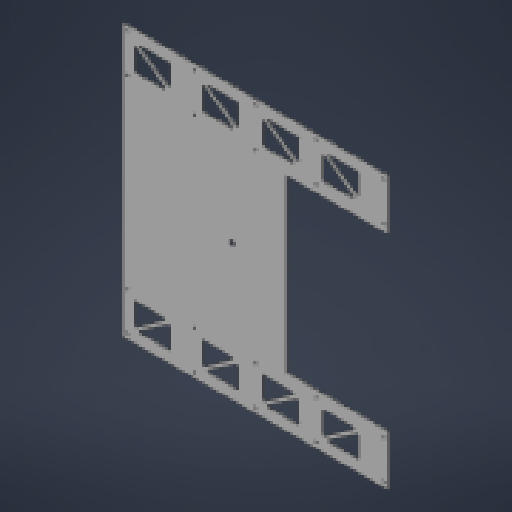
# Autodesk Inventor part: ВЕРХ 25-26
Saved by Autodesk Inventor 2026.2 (Build 302298000, 298)
## iProperties
Created: 2025-09-28
Part Number: ВЕРХ 25-26
Material: Типовые
Document SubType Name: Modeling
Designer: GameHD
Density: 1 g/cm^3
Appearance: По умолчанию
Author: GameHD
Autodesk Inventor part; units mm, degrees
ref_plane "YZ Plane" through (0, 0, 0) normal (1, 0, 0) x (0, 1, 0)
ref_plane "XZ Plane" through (0, 0, 0) normal (0, 1, 0) x (-1, 0, 0)
ref_plane "XY Plane" through (0, 0, 0) normal (0, 0, 1) x (1, 0, 0)
sketch "Эскиз1" plane through (0, 0, 0) normal (0, 0, 1) x (1, 0, 0)
  line L0 (0, 0) -> (380, 0)
  line L1 (380, 0) -> (380, 390)
  line L2 (380, 390) -> (0, 390)
  line L3 (0, 390) -> (0, 0)
  circle A0 centre (189.9999, 7.5) radius 1.625
  circle A1 centre (276.4236, 7.5) radius 1.625
  circle A2 centre (103.5763, 7.5) radius 1.625
  circle A3 centre (373.8998, 7.5) radius 1.625
  circle A4 centre (6.1, 7.5) radius 1.625
  circle A5 centre (964.1922, -67.5828) radius 2.1
  arc A6 (951.6923, -3.9328) -> (946.6923, -8.9328) centre (951.6923, -8.9328) ccw
  line L4 (0, -31.725) -> (0, 41.275)
  line L5 (1326.6922, -81.9328) -> (946.6923, -81.9328)
  line L6 (1326.6922, -8.9328) -> (1326.6922, -81.9328)
  arc A7 (1326.6922, -8.9328) -> (1321.6922, -3.9328) centre (1321.6922, -8.9328) ccw
  line L7 (951.6923, -3.9328) -> (1321.6922, -3.9328)
  line L8 (1216.76, -45.3471) -> (1194.7481, -38.048)
  arc A8 (1220.1863, -50.093) -> (1216.76, -45.3471) centre (1215.1863, -50.093) ccw
  line L9 (1220.1863, -56.3474) -> (1220.1863, -50.093)
  arc A9 (1215.4065, -61.3426) -> (1220.1863, -56.3474) centre (1215.1863, -56.3474) ccw
  line L10 (1169.4571, -63.3681) -> (1215.4065, -61.3426)
  arc A10 (1167.2037, -58.2497) -> (1169.4571, -63.3681) centre (1169.325, -60.3711) ccw
  line L11 (1187.1864, -40.5343) -> (1167.2037, -58.2497)
  arc A11 (1188.5574, -40.0313) -> (1187.1864, -40.5343) centre (1188.5132, -42.0308) ccw
  arc A12 (1188.5574, -40.0313) -> (1192.7788, -38.4615) centre (1188.6922, -33.9328) ccw
  arc A13 (1194.7481, -38.048) -> (1192.7788, -38.4615) centre (1194.1187, -39.9464) ccw
  circle A14 centre (1242.1863, -55.1828) radius 2.15
  circle A15 centre (1226.1863, -55.1828) radius 2.15
  circle A16 centre (1031.1982, -55.1828) radius 2.15
  line L12 (1053.1982, -50.093) -> (1053.1982, -56.3474)
  arc A17 (1056.6245, -45.3471) -> (1053.1982, -50.093) centre (1058.1982, -50.093) ccw
  line L13 (1078.6364, -38.048) -> (1056.6245, -45.3471)
  arc A18 (1080.6057, -38.4615) -> (1078.6364, -38.048) centre (1079.2659, -39.9464) ccw
  arc A19 (1080.6057, -38.4615) -> (1085.5622, -39.9705) centre (1084.6923, -33.9328) ccw
  line L14 (1106.1809, -58.2497) -> (1085.5622, -39.9705)
  arc A20 (1103.9274, -63.3681) -> (1106.1809, -58.2497) centre (1104.0595, -60.3711) ccw
  line L15 (1057.978, -61.3426) -> (1103.9274, -63.3681)
  arc A21 (1053.1982, -56.3474) -> (1057.978, -61.3426) centre (1058.1982, -56.3474) ccw
  circle A22 centre (1047.1982, -55.1828) radius 2.15
  circle A23 centre (1031.1982, -71.1828) radius 2.15
  circle A24 centre (1242.1863, -71.1828) radius 2.15
  circle A25 centre (1093.6922, -74.4328) radius 1.625
  circle A26 centre (1226.1863, -71.1828) radius 2.15
  circle A27 centre (1047.1982, -71.1828) radius 2.15
  circle A28 centre (1154.6923, -73.9328) radius 3.1
  line L16 (1209.2141, -15.9328) -> (1158.2349, -15.9328)
  arc A29 (1209.4653, -16.8651) -> (1209.2141, -15.9328) centre (1209.2141, -16.4328) ccw
  line L17 (1190.2429, -28.0332) -> (1209.4653, -16.8651)
  arc A30 (1190.2429, -28.0332) -> (1184.8228, -29.2171) centre (1188.6922, -33.9328) ccw
  arc A31 (1182.8362, -29.5377) -> (1184.8228, -29.2171) centre (1183.5541, -27.671) ccw
  line L18 (1157.517, -19.7995) -> (1182.8362, -29.5377)
  arc A32 (1158.2349, -15.9328) -> (1157.517, -19.7995) centre (1158.2349, -17.9328) ccw
  line L19 (1063.9192, -16.8651) -> (1083.1416, -28.0332)
  arc A33 (1064.1704, -15.9328) -> (1063.9192, -16.8651) centre (1064.1704, -16.4328) ccw
  line L20 (1115.1496, -15.9328) -> (1064.1704, -15.9328)
  arc A34 (1115.8675, -19.7995) -> (1115.1496, -15.9328) centre (1115.1496, -17.9328) ccw
  line L21 (1090.5483, -29.5377) -> (1115.8675, -19.7995)
  arc A35 (1088.5617, -29.2171) -> (1090.5483, -29.5377) centre (1089.8304, -27.671) ccw
  arc A36 (1088.5617, -29.2171) -> (1083.1416, -28.0332) centre (1084.6923, -33.9328) ccw
  line L22 (1110.9153, -57.1805) -> (1113.5672, -59.5315)
  arc A37 (1110.6057, -54.534) -> (1110.9153, -57.1805) centre (1112.2421, -55.6839) ccw
  line L23 (1131.0559, -25.4322) -> (1110.6057, -54.534)
  arc A38 (1134.6923, -26.5821) -> (1131.0559, -25.4322) centre (1132.6923, -26.5821) ccw
  line L24 (1134.6923, -61.3681) -> (1134.6923, -26.5821)
  arc A39 (1132.6923, -63.3681) -> (1134.6923, -61.3681) centre (1132.6923, -61.3681) ccw
  line L25 (1123.3837, -63.3681) -> (1132.6923, -63.3681)
  arc A40 (1121.7315, -62.4952) -> (1123.3837, -63.3681) centre (1123.3837, -61.3681) ccw
  arc A41 (1121.7315, -62.4952) -> (1115.338, -59.985) centre (1116.6923, -65.9328) ccw
  arc A42 (1113.5672, -59.5315) -> (1115.338, -59.985) centre (1114.894, -58.035) ccw
  line L26 (1168.4937, -51.8395) -> (1182.0952, -39.7813)
  arc A43 (1165.5306, -51.4929) -> (1168.4937, -51.8395) centre (1167.167, -50.343) ccw
  line L27 (1145.8825, -23.5324) -> (1165.5306, -51.4929)
  arc A44 (1148.2368, -20.5158) -> (1145.8825, -23.5324) centre (1147.5188, -22.3825) ccw
  line L28 (1180.7096, -33.0054) -> (1148.2368, -20.5158)
  arc A45 (1182.096, -34.0931) -> (1180.7096, -33.0054) centre (1179.6327, -35.8054) ccw
  arc A46 (1182.7689, -35.3904) -> (1182.096, -34.0931) centre (1177.4301, -37.3365) ccw
  arc A47 (1182.7689, -35.3904) -> (1182.9531, -35.9999) centre (1188.6922, -33.9328) ccw
  arc A48 (1183.0967, -37.7601) -> (1182.9531, -35.9999) centre (1177.4301, -37.3365) ccw
  arc A49 (1182.0952, -39.7813) -> (1183.0967, -37.7601) centre (1180.105, -37.5364) ccw
  line L29 (1125.1477, -20.5158) -> (1092.6749, -33.0054)
  arc A50 (1127.5021, -23.5324) -> (1125.1477, -20.5158) centre (1125.8657, -22.3825) ccw
  line L30 (1107.8539, -51.4929) -> (1127.5021, -23.5324)
  arc A51 (1104.8908, -51.8395) -> (1107.8539, -51.4929) centre (1106.2176, -50.343) ccw
  line L31 (1091.2893, -39.7813) -> (1104.8908, -51.8395)
  arc A52 (1090.2878, -37.7601) -> (1091.2893, -39.7813) centre (1093.2795, -37.5364) ccw
  arc A53 (1090.4314, -35.9999) -> (1090.2878, -37.7601) centre (1095.9544, -37.3365) ccw
  arc A54 (1090.4314, -35.9999) -> (1090.6156, -35.3904) centre (1084.6923, -33.9328) ccw
  arc A55 (1091.2885, -34.0931) -> (1090.6156, -35.3904) centre (1095.9544, -37.3365) ccw
  arc A56 (1092.6749, -33.0054) -> (1091.2885, -34.0931) centre (1093.7519, -35.8054) ccw
  line L32 (1162.7788, -54.534) -> (1142.3286, -25.4322)
  arc A57 (1162.4692, -57.1805) -> (1162.7788, -54.534) centre (1161.1424, -55.6839) ccw
  line L33 (1156.0575, -62.8647) -> (1162.4692, -57.1805)
  arc A58 (1154.7308, -63.3681) -> (1156.0575, -62.8647) centre (1154.7308, -61.3681) ccw
  line L34 (1140.6923, -63.3681) -> (1154.7308, -63.3681)
  arc A59 (1138.6923, -61.3681) -> (1140.6923, -63.3681) centre (1140.6923, -61.3681) ccw
  line L35 (1138.6923, -26.5821) -> (1138.6923, -61.3681)
  arc A60 (1142.3286, -25.4322) -> (1138.6923, -26.5821) centre (1140.6923, -26.5821) ccw
  arc A61 (1252.9105, -48.8923) -> (1251.6365, -50.9573) centre (1270.1159, -60.9328) ccw
  arc A62 (1249.247, -51.9056) -> (1251.6365, -50.9573) centre (1249.8765, -50.0073) ccw
  line L36 (1197.3221, -34.6874) -> (1249.247, -51.9056)
  arc A63 (1196.7592, -29.2459) -> (1197.3221, -34.6874) centre (1198.2663, -31.8398) ccw
  line L37 (1216.329, -17.8759) -> (1196.7592, -29.2459)
  arc A64 (1218.7614, -18.2046) -> (1216.329, -17.8759) centre (1217.3337, -19.6052) ccw
  arc A65 (1218.7614, -18.2046) -> (1224.7366, -19.8136) centre (1223.1159, -13.9328) ccw
  arc A66 (1226.6821, -20.3275) -> (1224.7366, -19.8136) centre (1225.2679, -21.7417) ccw
  line L38 (1252.6861, -46.3314) -> (1226.6821, -20.3275)
  arc A67 (1252.9105, -48.8923) -> (1252.6861, -46.3314) centre (1251.2719, -47.7456) ccw
  arc A68 (1048.648, -19.8136) -> (1054.6231, -18.2046) centre (1050.2686, -13.9328) ccw
  arc A69 (1057.0555, -17.8759) -> (1054.6231, -18.2046) centre (1056.0508, -19.6052) ccw
  line L39 (1076.6253, -29.2459) -> (1057.0555, -17.8759)
  arc A70 (1076.0624, -34.6874) -> (1076.6253, -29.2459) centre (1075.1182, -31.8398) ccw
  line L40 (1024.1375, -51.9056) -> (1076.0624, -34.6874)
  arc A71 (1021.7481, -50.9573) -> (1024.1375, -51.9056) centre (1023.508, -50.0073) ccw
  arc A72 (1021.7481, -50.9573) -> (1020.4741, -48.8923) centre (1003.2686, -60.9328) ccw
  arc A73 (1020.6985, -46.3314) -> (1020.4741, -48.8923) centre (1022.1127, -47.7456) ccw
  line L41 (1046.7024, -20.3275) -> (1020.6985, -46.3314)
  arc A74 (1048.648, -19.8136) -> (1046.7024, -20.3275) centre (1048.1166, -21.7417) ccw
  circle A75 centre (1039.1982, -63.1828) radius 6
  circle A76 centre (1234.1863, -63.1828) radius 6
  arc A77 (1291.0993, -61.7677) -> (1287.7395, -49.5132) centre (1270.1159, -60.9328) ccw
  arc A78 (1288.0551, -46.9619) -> (1287.7395, -49.5132) centre (1289.418, -48.4256) ccw
  line L42 (1313.5478, -23.2248) -> (1288.0551, -46.9619)
  arc A79 (1318.5922, -25.4204) -> (1313.5478, -23.2248) centre (1315.5922, -25.4204) ccw
  line L43 (1318.5922, -64.0897) -> (1318.5922, -25.4204)
  arc A80 (1318.0461, -65.8154) -> (1318.5922, -64.0897) centre (1315.5922, -64.0897) ccw
  arc A81 (1315.1572, -68.1426) -> (1318.0461, -65.8154) centre (1312.5518, -61.9515) ccw
  arc A82 (1313.3548, -68.3086) -> (1315.1572, -68.1426) centre (1313.9935, -65.3774) ccw
  line L44 (1292.6719, -63.8013) -> (1313.3548, -68.3086)
  arc A83 (1291.0993, -61.7677) -> (1292.6719, -63.8013) centre (1293.0977, -61.8472) ccw
  arc A84 (1015.3091, -43.7274) -> (990.6226, -44.1674) centre (1003.2686, -60.9328) ccw
  arc A85 (988.0553, -44.0344) -> (990.6226, -44.1674) centre (989.4182, -42.5707) ccw
  line L45 (963.455, -21.1284) -> (988.0553, -44.0344)
  arc A86 (965.4994, -15.9328) -> (963.455, -21.1284) centre (965.4994, -18.9328) ccw
  line L46 (1043.026, -15.9328) -> (965.4994, -15.9328)
  arc A87 (1043.7331, -17.6399) -> (1043.026, -15.9328) centre (1043.026, -16.9328) ccw
  line L47 (1017.87, -43.503) -> (1043.7331, -17.6399)
  arc A88 (1015.3091, -43.7274) -> (1017.87, -43.503) centre (1016.4558, -42.0887) ccw
  line L48 (1229.6514, -17.6399) -> (1255.5145, -43.503)
  arc A89 (1230.3585, -15.9328) -> (1229.6514, -17.6399) centre (1230.3585, -16.9328) ccw
  line L49 (1307.8851, -15.9328) -> (1230.3585, -15.9328)
  arc A90 (1309.9295, -21.1284) -> (1307.8851, -15.9328) centre (1307.8851, -18.9328) ccw
  line L50 (1285.3292, -44.0344) -> (1309.9295, -21.1284)
  arc A91 (1282.7619, -44.1674) -> (1285.3292, -44.0344) centre (1283.9663, -42.5707) ccw
  arc A92 (1282.7619, -44.1674) -> (1258.0754, -43.7274) centre (1270.1159, -60.9328) ccw
  arc A93 (1255.5145, -43.503) -> (1258.0754, -43.7274) centre (1256.9287, -42.0887) ccw
  circle A94 centre (1319.6922, -74.4328) radius 1.625
  circle A95 centre (953.6923, -74.4328) radius 1.625
  circle A96 centre (1179.6922, -74.4328) radius 1.625
  circle A97 centre (1084.6923, -33.9328) radius 2.1
  circle A98 centre (1116.6923, -65.9328) radius 2.1
  circle A99 centre (1003.2686, -60.9328) radius 4
  circle A100 centre (994.2686, -60.9328) radius 2.1
  circle A101 centre (1279.1159, -60.9328) radius 2.1
  circle A102 centre (1270.1159, -69.9328) radius 2.1
  circle A103 centre (1270.1159, -60.9328) radius 4
  circle A104 centre (1003.2686, -51.9328) radius 2.1
  circle A105 centre (1003.2686, -69.9328) radius 2.1
  circle A106 centre (1012.2686, -60.9328) radius 2.1
  circle A107 centre (1270.1159, -51.9328) radius 2.1
  circle A108 centre (1261.1159, -60.9328) radius 2.1
  arc A109 (969.1578, -64.2135) -> (967.1922, -62.5828) centre (967.1922, -64.5828) ccw
  line L51 (967.1922, -62.5828) -> (956.7923, -62.5828)
  arc A110 (954.7923, -60.5828) -> (956.7923, -62.5828) centre (956.7923, -60.5828) ccw
  line L52 (954.7923, -25.4204) -> (954.7923, -60.5828)
  arc A111 (959.8367, -23.2248) -> (954.7923, -25.4204) centre (957.7923, -25.4204) ccw
  line L53 (985.3295, -46.9619) -> (959.8367, -23.2248)
  arc A112 (985.645, -49.5132) -> (985.3295, -46.9619) centre (983.9666, -48.4256) ccw
  arc A113 (985.645, -49.5132) -> (982.2852, -61.7677) centre (1003.2686, -60.9328) ccw
  arc A114 (980.7127, -63.8013) -> (982.2852, -61.7677) centre (980.2868, -61.8472) ccw
  line L54 (971.5492, -65.7983) -> (980.7127, -63.8013)
  arc A115 (969.1578, -64.2135) -> (971.5492, -65.7983) centre (971.1234, -63.8441) ccw
  line L55 (0, 195) -> (417.5125, 195)
  circle A116 centre (189.9999, 382.5) radius 1.625
  circle A117 centre (276.4236, 382.5) radius 1.625
  circle A118 centre (373.8998, 382.5) radius 1.625
  circle A119 centre (103.5763, 382.5) radius 1.625
  circle A120 centre (6.1, 382.5) radius 1.625
  line L56 (-36.5125, 35) -> (652.4625, 35)
  circle A121 centre (189.9999, 62.5) radius 1.625
  circle A122 centre (276.4236, 62.5) radius 1.625
  circle A123 centre (373.8998, 62.5) radius 1.625
  circle A124 centre (103.5763, 62.5) radius 1.625
  circle A125 centre (6.1, 62.5) radius 1.625
  circle A126 centre (189.9999, 327.5) radius 1.625
  circle A127 centre (103.5763, 327.5) radius 1.625
  circle A128 centre (373.8998, 327.5) radius 1.625
  circle A129 centre (6.1, 327.5) radius 1.625
  circle A130 centre (276.4236, 327.5) radius 1.625
  line L57 (380, 195) -> (280, 195)
  line L58 (280, 195) -> (280, 73)
  line L59 (280, 73) -> (380, 73)
  line L60 (380, 73) -> (380, 195)
  line L61 (280, 195) -> (280, 317)
  line L62 (280, 317) -> (380, 317)
  point P0 (1137.8297, -60.6207)
  point P1 (0, 348.725)
  dimension "d0" = 380
  dimension "d1" = 390
  dimension "d2" = 7.5
  dimension "d3" = 0
  dimension "d4" = 0
  dimension "d5" = 0
  dimension "d6" = 0
  dimension "d7" = 35
  dimension "d8" = 100
  dimension "d9" = 122
  constraints: 166 point on circle, 131 centre point, 126 end point, 18 symmetric about line, 4 horizontal, 4 parallel, 2 midpoint, 2 perpendicular, 1 point on line, 15 other
  measures "d0" distance of L2.end L1.end
  measures "d1" distance of L1.end L0.end
  measures "d2" distance from line of L0 A4.centre
  measures "d3" vertical distance of A4.centre A2.centre
  measures "d4" vertical distance of A2.centre A0.centre
  measures "d5" vertical distance of A0.centre A1.centre
  measures "d6" vertical distance of A1.centre A3.centre
  measures "d7" distance between parallel lines of L0 L56
  measures "d8" distance of L59.end L58.end
  measures "d9" distance of L58.end L57.end
extrude "Выдавливание1" add sketch "Эскиз1" along normal blind 1.5 contours L3 L56 L1 L0 | L3 L55 L58 L59 L1 L56 | L3 L2 L1 L62 L61 L55
sketch "Эскиз2" plane through (0, 0, 1.5) normal (0, 0, 1) x (1, 0, 0)
  line L0 (25.7748, 373.5) -> (65.85, 373.5)
  arc A0 (67.85, 371.5) -> (65.85, 373.5) centre (65.85, 371.5) ccw
  arc A1 (25.7748, 373.5) -> (24.6115, 369.8731) centre (25.7748, 371.5) ccw
  arc A2 (19.2632, 368.7798) -> (16.1, 367.1528) centre (18.1, 367.1528) ccw
  line L1 (67.85, 371.5) -> (67.85, 344.5882)
  line L2 (64.6868, 342.9612) -> (24.6115, 369.8731)
  line L3 (67.85, 336.5) -> (16.1, 373.5)
  arc A3 (58.1752, 336.5) -> (59.3385, 340.1269) centre (58.1752, 338.5) ccw
  arc A4 (64.6868, 342.9612) -> (67.85, 344.5882) centre (65.85, 344.5882) ccw
  line L4 (58.1752, 336.5) -> (18.1, 336.5)
  line L5 (16.1, 338.5) -> (16.1, 367.1528)
  arc A5 (16.1, 338.5) -> (18.1, 336.5) centre (18.1, 338.5) ccw
  line L6 (59.3385, 340.1269) -> (19.2632, 368.7798)
  circle A6 centre (6.1, 382.5) radius 1.625 projected
  line L7 (280, 73) -> (280, 317) projected
  line L8 (280, 317) -> (380, 317) projected
  line L9 (380, 317) -> (380, 390) projected
  line L10 (380, 390) -> (0, 390) projected
  line L11 (0, 390) -> (0, 0) projected
  line L12 (0, 0) -> (380, 0) projected
  line L13 (380, 0) -> (380, 73) projected
  line L14 (380, 73) -> (280, 73) projected
  circle A7 centre (373.8998, 327.5) radius 1.625 projected
  circle A8 centre (189.9999, 327.5) radius 1.625 projected
  circle A9 centre (6.1, 327.5) radius 1.625 projected
  circle A10 centre (103.5763, 382.5) radius 1.625 projected
  circle A11 centre (276.4236, 382.5) radius 1.625 projected
  circle A12 centre (189.9999, 382.5) radius 1.625 projected
  circle A13 centre (373.8998, 382.5) radius 1.625 projected
  circle A14 centre (6.1, 382.5) radius 1.625 projected
  circle A15 centre (103.5763, 327.5) radius 1.625 projected
  circle A16 centre (276.4236, 327.5) radius 1.625 projected
  circle A17 centre (103.5763, 7.5) radius 1.625 projected
  circle A18 centre (373.8998, 7.5) radius 1.625 projected
  circle A19 centre (276.4236, 7.5) radius 1.625 projected
  circle A20 centre (189.9999, 7.5) radius 1.625 projected
  circle A21 centre (6.1, 7.5) radius 1.625 projected
  circle A22 centre (189.9999, 62.5) radius 1.625 projected
  circle A23 centre (103.5763, 62.5) radius 1.625 projected
  circle A24 centre (373.8998, 62.5) radius 1.625 projected
  circle A25 centre (6.1, 62.5) radius 1.625 projected
  circle A26 centre (276.4236, 62.5) radius 1.625 projected
  arc A27 (123.251, 373.5) -> (122.0878, 369.8731) centre (123.251, 371.5) ccw
  arc A28 (116.7395, 368.7798) -> (113.5763, 367.1528) centre (115.5763, 367.1528) ccw
  line L15 (113.5763, 338.5) -> (113.5763, 367.1528)
  arc A29 (113.5763, 338.5) -> (115.5763, 336.5) centre (115.5763, 338.5) ccw
  line L16 (123.251, 373.5) -> (163.3263, 373.5)
  line L17 (156.8147, 340.1269) -> (116.7395, 368.7798)
  line L18 (155.6515, 336.5) -> (115.5763, 336.5)
  line L19 (165.3263, 336.5) -> (113.5763, 373.5)
  line L20 (162.1631, 342.9612) -> (122.0878, 369.8731)
  arc A30 (165.3263, 371.5) -> (163.3263, 373.5) centre (163.3263, 371.5) ccw
  line L21 (165.3263, 371.5) -> (165.3263, 344.5882)
  arc A31 (155.6515, 336.5) -> (156.8147, 340.1269) centre (155.6515, 338.5) ccw
  arc A32 (162.1631, 342.9612) -> (165.3263, 344.5882) centre (163.3263, 344.5882) ccw
  arc A33 (209.6747, 373.5) -> (208.5115, 369.8731) centre (209.6747, 371.5) ccw
  arc A34 (203.1631, 368.7798) -> (199.9999, 367.1528) centre (201.9999, 367.1528) ccw
  line L22 (199.9999, 338.5) -> (199.9999, 367.1528)
  arc A35 (199.9999, 338.5) -> (201.9999, 336.5) centre (201.9999, 338.5) ccw
  line L23 (209.6747, 373.5) -> (249.7499, 373.5)
  line L24 (243.2384, 340.1269) -> (203.1631, 368.7798)
  line L25 (242.0752, 336.5) -> (201.9999, 336.5)
  line L26 (251.7499, 336.5) -> (199.9999, 373.5)
  line L27 (248.5867, 342.9612) -> (208.5115, 369.8731)
  arc A36 (251.7499, 371.5) -> (249.7499, 373.5) centre (249.7499, 371.5) ccw
  line L28 (251.7499, 371.5) -> (251.7499, 344.5882)
  arc A37 (242.0752, 336.5) -> (243.2384, 340.1269) centre (242.0752, 338.5) ccw
  arc A38 (248.5867, 342.9612) -> (251.7499, 344.5882) centre (249.7499, 344.5882) ccw
  arc A39 (296.0983, 373.5) -> (294.9351, 369.8731) centre (296.0983, 371.5) ccw
  arc A40 (289.5868, 368.7798) -> (286.4236, 367.1528) centre (288.4236, 367.1528) ccw
  line L29 (286.4236, 338.5) -> (286.4236, 367.1528)
  arc A41 (286.4236, 338.5) -> (288.4236, 336.5) centre (288.4236, 338.5) ccw
  line L30 (296.0983, 373.5) -> (336.1736, 373.5)
  line L31 (329.662, 340.1269) -> (289.5868, 368.7798)
  line L32 (328.4988, 336.5) -> (288.4236, 336.5)
  line L33 (338.1736, 336.5) -> (286.4236, 373.5)
  line L34 (335.0103, 342.9612) -> (294.9351, 369.8731)
  arc A42 (338.1736, 371.5) -> (336.1736, 373.5) centre (336.1736, 371.5) ccw
  line L35 (338.1736, 371.5) -> (338.1736, 344.5882)
  arc A43 (328.4988, 336.5) -> (329.662, 340.1269) centre (328.4988, 338.5) ccw
  arc A44 (335.0103, 342.9612) -> (338.1736, 344.5882) centre (336.1736, 344.5882) ccw
  line L36 (0, 195) -> (395.2875, 195)
  arc A45 (24.6115, 20.1269) -> (25.7748, 16.5) centre (25.7748, 18.5) ccw
  arc A46 (16.1, 22.8472) -> (19.2632, 21.2202) centre (18.1, 22.8472) ccw
  line L37 (16.1, 51.5) -> (16.1, 22.8472)
  arc A47 (18.1, 53.5) -> (16.1, 51.5) centre (18.1, 51.5) ccw
  line L38 (25.7748, 16.5) -> (65.85, 16.5)
  line L39 (59.3385, 49.8731) -> (19.2632, 21.2202)
  line L40 (58.1752, 53.5) -> (18.1, 53.5)
  line L41 (67.85, 53.5) -> (16.1, 16.5)
  line L42 (64.6868, 47.0388) -> (24.6115, 20.1269)
  arc A48 (65.85, 16.5) -> (67.85, 18.5) centre (65.85, 18.5) ccw
  line L43 (67.85, 18.5) -> (67.85, 45.4118)
  arc A49 (59.3385, 49.8731) -> (58.1752, 53.5) centre (58.1752, 51.5) ccw
  arc A50 (67.85, 45.4118) -> (64.6868, 47.0388) centre (65.85, 45.4118) ccw
  line L44 (155.6515, 53.5) -> (115.5763, 53.5)
  line L45 (156.8147, 49.8731) -> (116.7395, 21.2202)
  line L46 (165.3263, 53.5) -> (113.5763, 16.5)
  line L47 (162.1631, 47.0388) -> (122.0878, 20.1269)
  arc A51 (156.8147, 49.8731) -> (155.6515, 53.5) centre (155.6515, 51.5) ccw
  arc A52 (165.3263, 45.4118) -> (162.1631, 47.0388) centre (163.3263, 45.4118) ccw
  line L48 (165.3263, 18.5) -> (165.3263, 45.4118)
  arc A53 (163.3263, 16.5) -> (165.3263, 18.5) centre (163.3263, 18.5) ccw
  line L49 (123.251, 16.5) -> (163.3263, 16.5)
  arc A54 (115.5763, 53.5) -> (113.5763, 51.5) centre (115.5763, 51.5) ccw
  arc A55 (122.0878, 20.1269) -> (123.251, 16.5) centre (123.251, 18.5) ccw
  line L50 (113.5763, 51.5) -> (113.5763, 22.8472)
  arc A56 (113.5763, 22.8472) -> (116.7395, 21.2202) centre (115.5763, 22.8472) ccw
  line L51 (242.0752, 53.5) -> (201.9999, 53.5)
  line L52 (243.2384, 49.8731) -> (203.1631, 21.2202)
  line L53 (251.7499, 53.5) -> (199.9999, 16.5)
  line L54 (248.5867, 47.0388) -> (208.5115, 20.1269)
  arc A57 (243.2384, 49.8731) -> (242.0752, 53.5) centre (242.0752, 51.5) ccw
  arc A58 (251.7499, 45.4118) -> (248.5867, 47.0388) centre (249.7499, 45.4118) ccw
  line L55 (251.7499, 18.5) -> (251.7499, 45.4118)
  arc A59 (249.7499, 16.5) -> (251.7499, 18.5) centre (249.7499, 18.5) ccw
  line L56 (209.6747, 16.5) -> (249.7499, 16.5)
  arc A60 (201.9999, 53.5) -> (199.9999, 51.5) centre (201.9999, 51.5) ccw
  arc A61 (208.5115, 20.1269) -> (209.6747, 16.5) centre (209.6747, 18.5) ccw
  line L57 (199.9999, 51.5) -> (199.9999, 22.8472)
  arc A62 (199.9999, 22.8472) -> (203.1631, 21.2202) centre (201.9999, 22.8472) ccw
  line L58 (328.4988, 53.5) -> (288.4236, 53.5)
  line L59 (329.662, 49.8731) -> (289.5868, 21.2202)
  line L60 (338.1736, 53.5) -> (286.4236, 16.5)
  line L61 (335.0103, 47.0388) -> (294.9351, 20.1269)
  arc A63 (329.662, 49.8731) -> (328.4988, 53.5) centre (328.4988, 51.5) ccw
  arc A64 (338.1736, 45.4118) -> (335.0103, 47.0388) centre (336.1736, 45.4118) ccw
  line L62 (338.1736, 18.5) -> (338.1736, 45.4118)
  arc A65 (336.1736, 16.5) -> (338.1736, 18.5) centre (336.1736, 18.5) ccw
  line L63 (296.0983, 16.5) -> (336.1736, 16.5)
  arc A66 (288.4236, 53.5) -> (286.4236, 51.5) centre (288.4236, 51.5) ccw
  arc A67 (294.9351, 20.1269) -> (296.0983, 16.5) centre (296.0983, 18.5) ccw
  line L64 (286.4236, 51.5) -> (286.4236, 22.8472)
  arc A68 (286.4236, 22.8472) -> (289.5868, 21.2202) centre (288.4236, 22.8472) ccw
  dimension "d12" = 37
  dimension "d13" = 51.75
  dimension "d16" = 10
  dimension "d17" = 9
  dimension "d18" = 47.75
  dimension "d19" = 4.3472
  dimension "d20" = 33
  dimension "d21" = 2
  dimension "d22" = 2
  dimension "d23" = 2
  dimension "d24" = 2
  dimension "d25" = 2
  dimension "d26" = 2
  dimension "d27" = 28.6528
  dimension "d28" = 2
  dimension "d29" = 37
  dimension "d30" = 51.75
  dimension "d31" = 47.75
  dimension "d32" = 4.3472
  dimension "d33" = 33
  dimension "d34" = 2
  dimension "d35" = 2
  dimension "d36" = 2
  dimension "d37" = 2
  dimension "d38" = 2
  dimension "d39" = 2
  dimension "d40" = 28.6528
  dimension "d41" = 2
  dimension "d42" = 37
  dimension "d43" = 51.75
  dimension "d44" = 47.75
  dimension "d45" = 4.3472
  dimension "d46" = 33
  dimension "d47" = 2
  dimension "d48" = 2
  dimension "d49" = 2
  dimension "d50" = 2
  dimension "d51" = 2
  dimension "d52" = 2
  dimension "d53" = 28.6528
  dimension "d54" = 2
  dimension "d55" = 37
  dimension "d56" = 51.75
  dimension "d57" = 47.75
  dimension "d58" = 4.3472
  dimension "d59" = 33
  dimension "d60" = 2
  dimension "d61" = 2
  dimension "d62" = 2
  dimension "d63" = 2
  dimension "d64" = 2
  dimension "d65" = 2
  dimension "d66" = 28.6528
  dimension "d67" = 2
  constraints: 114 end point, 96 point on circle, 80 symmetric about line, 48 centre point, 32 point on line, 1 horizontal, 1 midpoint, 24 other
  measures "d12" distance between parallel lines of L4 L0
  measures "d13" distance between parallel lines of L1 L5
  measures "d16" distance from line of A6.centre L5
  measures "d17" distance from line of A6.centre L0
  measures "d18" horizontal distance of A0.centre A5.centre
  measures "d19" vertical distance of A1.centre A2.centre
  measures "d20" vertical distance of A3.centre A1.centre
  measures "d21" radius of A1
  measures "d22" radius of A2
  measures "d23" radius of A5
  measures "d24" radius of A3
  measures "d25" radius of A0
  measures "d26" radius of A4
  measures "d27" distance of L5.start L5.end
  measures "d28" distance from line of A2.centre L5
  measures "d29" distance between parallel lines of L18 L16
  measures "d30" distance between parallel lines of L21 L15
  measures "d31" horizontal distance of A30.centre A29.centre
  measures "d32" vertical distance of A27.centre A28.centre
  measures "d33" vertical distance of A31.centre A27.centre
  measures "d34" radius of A27
  measures "d35" radius of A28
  measures "d36" radius of A29
  measures "d37" radius of A31
  measures "d38" radius of A30
  measures "d39" radius of A32
  measures "d40" distance of L15.start L15.end
  measures "d41" distance from line of A28.centre L15
  measures "d42" distance between parallel lines of L25 L23
  measures "d43" distance between parallel lines of L28 L22
  measures "d44" horizontal distance of A36.centre A35.centre
  measures "d45" vertical distance of A33.centre A34.centre
  measures "d46" vertical distance of A37.centre A33.centre
  measures "d47" radius of A33
  measures "d48" radius of A34
  measures "d49" radius of A35
  measures "d50" radius of A37
  measures "d51" radius of A36
  measures "d52" radius of A38
  measures "d53" distance of L22.start L22.end
  measures "d54" distance from line of A34.centre L22
  measures "d55" distance between parallel lines of L32 L30
  measures "d56" distance between parallel lines of L35 L29
  measures "d57" horizontal distance of A42.centre A41.centre
  measures "d58" vertical distance of A39.centre A40.centre
  measures "d59" vertical distance of A43.centre A39.centre
  measures "d60" radius of A39
  measures "d61" radius of A40
  measures "d62" radius of A41
  measures "d63" radius of A43
  measures "d64" radius of A42
  measures "d65" radius of A44
  measures "d66" distance of L29.start L29.end
  measures "d67" distance from line of A40.centre L29
extrude "Выдавливание2" cut sketch "Эскиз2" against normal blind 1.5 contours L0 A0 L1 A4 L2 A1 | L6 A3 L4 A5 L5 A2 | L16 A30 L21 A32 L20 A27 | L17 A31 L18 A29 L15 A28 | L23 A36 L28 A38 L27 A33 | L24 A37 L25 A35 L22 A34 | L30 A42 L35 A44 L34 A39 | L31 A43 L32 A41 L29 A40 | L42 A50 L43 A48 L38 A45 | L37 A47 L40 A49 L39 A46 | A51 L45 A56 L50 A54 L44 | A52 L48 A53 L49 A55 L47 | A57 L52 A62 L57 A60 L51 | A58 L55 A59 L56 A61 L54 | A63 L59 A68 L64 A66 L58 | A64 L62 A65 L63 A67 L61
sketch "Эскиз4" plane through (0, 0, 1.5) normal (0, 0, 1) x (1, 0, 0)
  line L0 (391.3464, 129.9271) -> (391.3464, 259.9271) projected
  line L1 (199.3064, 259.9271) -> (391.3464, 259.9271) projected
  line L2 (199.3064, 129.9271) -> (199.3064, 259.9271) projected
  line L3 (391.3464, 129.9271) -> (199.3064, 129.9271) projected
  circle A0 centre (276.4236, 62.5) radius 1.625 projected
  circle A1 centre (6.1, 62.5) radius 1.625 projected
  circle A2 centre (373.8998, 62.5) radius 1.625 projected
  circle A3 centre (103.5763, 62.5) radius 1.625 projected
  circle A4 centre (189.9999, 62.5) radius 1.625 projected
  circle A5 centre (6.1, 7.5) radius 1.625 projected
  circle A6 centre (189.9999, 7.5) radius 1.625 projected
  circle A7 centre (276.4236, 7.5) radius 1.625 projected
  circle A8 centre (373.8998, 7.5) radius 1.625 projected
  circle A9 centre (103.5763, 7.5) radius 1.625 projected
  circle A10 centre (276.4236, 327.5) radius 1.625 projected
  circle A11 centre (103.5763, 327.5) radius 1.625 projected
  circle A12 centre (6.1, 382.5) radius 1.625 projected
  circle A13 centre (373.8998, 382.5) radius 1.625 projected
  circle A14 centre (189.9999, 382.5) radius 1.625 projected
  circle A15 centre (276.4236, 382.5) radius 1.625 projected
  circle A16 centre (103.5763, 382.5) radius 1.625 projected
  circle A17 centre (6.1, 327.5) radius 1.625 projected
  circle A18 centre (189.9999, 327.5) radius 1.625 projected
  circle A19 centre (373.8998, 327.5) radius 1.625 projected
  line L4 (0, 390) -> (0, 0) projected
  line L5 (0, 0) -> (380, 0) projected
  line L6 (380, 0) -> (380, 73) projected
  line L7 (380, 73) -> (280, 73) projected
  line L8 (280, 73) -> (280, 317) projected
  line L9 (280, 317) -> (380, 317) projected
  line L10 (380, 317) -> (380, 390) projected
  line L11 (380, 390) -> (0, 390) projected
  line L12 (67.85, 45.4118) -> (67.85, 18.5) projected
  arc A20 (65.85, 16.5) -> (67.85, 18.5) centre (65.85, 18.5) ccw projected
  line L13 (65.85, 16.5) -> (25.7748, 16.5) projected
  arc A21 (24.6115, 20.1269) -> (25.7748, 16.5) centre (25.7748, 18.5) ccw projected
  line L14 (24.6115, 20.1269) -> (64.6868, 47.0388) projected
  arc A22 (67.85, 45.4118) -> (64.6868, 47.0388) centre (65.85, 45.4118) ccw projected
  arc A23 (201.9999, 53.5) -> (199.9999, 51.5) centre (201.9999, 51.5) ccw projected
  line L15 (201.9999, 53.5) -> (242.0752, 53.5) projected
  arc A24 (243.2384, 49.8731) -> (242.0752, 53.5) centre (242.0752, 51.5) ccw projected
  line L16 (243.2384, 49.8731) -> (203.1631, 21.2202) projected
  arc A25 (199.9999, 22.8472) -> (203.1631, 21.2202) centre (201.9999, 22.8472) ccw projected
  line L17 (199.9999, 22.8472) -> (199.9999, 51.5) projected
  arc A26 (25.7748, 373.5) -> (24.6115, 369.8731) centre (25.7748, 371.5) ccw projected
  line L18 (25.7748, 373.5) -> (65.85, 373.5) projected
  arc A27 (67.85, 371.5) -> (65.85, 373.5) centre (65.85, 371.5) ccw projected
  line L19 (67.85, 371.5) -> (67.85, 344.5882) projected
  arc A28 (64.6868, 342.9612) -> (67.85, 344.5882) centre (65.85, 344.5882) ccw projected
  line L20 (64.6868, 342.9612) -> (24.6115, 369.8731) projected
  line L21 (199.9999, 338.5) -> (199.9999, 367.1528) projected
  arc A29 (203.1631, 368.7798) -> (199.9999, 367.1528) centre (201.9999, 367.1528) ccw projected
  line L22 (203.1631, 368.7798) -> (243.2384, 340.1269) projected
  arc A30 (242.0752, 336.5) -> (243.2384, 340.1269) centre (242.0752, 338.5) ccw projected
  line L23 (242.0752, 336.5) -> (201.9999, 336.5) projected
  arc A31 (199.9999, 338.5) -> (201.9999, 336.5) centre (201.9999, 338.5) ccw projected
  arc A32 (296.0983, 373.5) -> (294.9351, 369.8731) centre (296.0983, 371.5) ccw projected
  line L24 (296.0983, 373.5) -> (336.1736, 373.5) projected
  arc A33 (338.1736, 371.5) -> (336.1736, 373.5) centre (336.1736, 371.5) ccw projected
  line L25 (338.1736, 371.5) -> (338.1736, 344.5882) projected
  arc A34 (335.0103, 342.9612) -> (338.1736, 344.5882) centre (336.1736, 344.5882) ccw projected
  line L26 (335.0103, 342.9612) -> (294.9351, 369.8731) projected
  arc A35 (123.251, 373.5) -> (122.0878, 369.8731) centre (123.251, 371.5) ccw projected
  line L27 (123.251, 373.5) -> (163.3263, 373.5) projected
  arc A36 (165.3263, 371.5) -> (163.3263, 373.5) centre (163.3263, 371.5) ccw projected
  line L28 (165.3263, 371.5) -> (165.3263, 344.5882) projected
  arc A37 (162.1631, 342.9612) -> (165.3263, 344.5882) centre (163.3263, 344.5882) ccw projected
  line L29 (162.1631, 342.9612) -> (122.0878, 369.8731) projected
  arc A38 (336.1736, 16.5) -> (338.1736, 18.5) centre (336.1736, 18.5) ccw projected
  line L30 (336.1736, 16.5) -> (296.0983, 16.5) projected
  arc A39 (294.9351, 20.1269) -> (296.0983, 16.5) centre (296.0983, 18.5) ccw projected
  line L31 (294.9351, 20.1269) -> (335.0103, 47.0388) projected
  arc A40 (338.1736, 45.4118) -> (335.0103, 47.0388) centre (336.1736, 45.4118) ccw projected
  line L32 (338.1736, 45.4118) -> (338.1736, 18.5) projected
  arc A41 (122.0878, 20.1269) -> (123.251, 16.5) centre (123.251, 18.5) ccw projected
  line L33 (122.0878, 20.1269) -> (162.1631, 47.0388) projected
  arc A42 (165.3263, 45.4118) -> (162.1631, 47.0388) centre (163.3263, 45.4118) ccw projected
  line L34 (165.3263, 45.4118) -> (165.3263, 18.5) projected
  arc A43 (163.3263, 16.5) -> (165.3263, 18.5) centre (163.3263, 18.5) ccw projected
  line L35 (163.3263, 16.5) -> (123.251, 16.5) projected
  line L36 (16.1, 22.8472) -> (16.1, 51.5) projected
  arc A44 (18.1, 53.5) -> (16.1, 51.5) centre (18.1, 51.5) ccw projected
  line L37 (18.1, 53.5) -> (58.1752, 53.5) projected
  arc A45 (59.3385, 49.8731) -> (58.1752, 53.5) centre (58.1752, 51.5) ccw projected
  line L38 (59.3385, 49.8731) -> (19.2632, 21.2202) projected
  arc A46 (16.1, 22.8472) -> (19.2632, 21.2202) centre (18.1, 22.8472) ccw projected
  arc A47 (249.7499, 16.5) -> (251.7499, 18.5) centre (249.7499, 18.5) ccw projected
  line L39 (249.7499, 16.5) -> (209.6747, 16.5) projected
  arc A48 (208.5115, 20.1269) -> (209.6747, 16.5) centre (209.6747, 18.5) ccw projected
  line L40 (208.5115, 20.1269) -> (248.5867, 47.0388) projected
  arc A49 (251.7499, 45.4118) -> (248.5867, 47.0388) centre (249.7499, 45.4118) ccw projected
  line L41 (251.7499, 45.4118) -> (251.7499, 18.5) projected
  arc A50 (19.2632, 368.7798) -> (16.1, 367.1528) centre (18.1, 367.1528) ccw projected
  line L42 (19.2632, 368.7798) -> (59.3385, 340.1269) projected
  arc A51 (58.1752, 336.5) -> (59.3385, 340.1269) centre (58.1752, 338.5) ccw projected
  line L43 (58.1752, 336.5) -> (18.1, 336.5) projected
  arc A52 (16.1, 338.5) -> (18.1, 336.5) centre (18.1, 338.5) ccw projected
  line L44 (16.1, 338.5) -> (16.1, 367.1528) projected
  arc A53 (209.6747, 373.5) -> (208.5115, 369.8731) centre (209.6747, 371.5) ccw projected
  line L45 (209.6747, 373.5) -> (249.7499, 373.5) projected
  arc A54 (251.7499, 371.5) -> (249.7499, 373.5) centre (249.7499, 371.5) ccw projected
  line L46 (251.7499, 371.5) -> (251.7499, 344.5882) projected
  arc A55 (248.5867, 342.9612) -> (251.7499, 344.5882) centre (249.7499, 344.5882) ccw projected
  line L47 (248.5867, 342.9612) -> (208.5115, 369.8731) projected
  line L48 (286.4236, 338.5) -> (286.4236, 367.1528) projected
  arc A56 (289.5868, 368.7798) -> (286.4236, 367.1528) centre (288.4236, 367.1528) ccw projected
  line L49 (289.5868, 368.7798) -> (329.662, 340.1269) projected
  arc A57 (328.4988, 336.5) -> (329.662, 340.1269) centre (328.4988, 338.5) ccw projected
  line L50 (328.4988, 336.5) -> (288.4236, 336.5) projected
  arc A58 (286.4236, 338.5) -> (288.4236, 336.5) centre (288.4236, 338.5) ccw projected
  line L51 (113.5763, 338.5) -> (113.5763, 367.1528) projected
  arc A59 (116.7395, 368.7798) -> (113.5763, 367.1528) centre (115.5763, 367.1528) ccw projected
  line L52 (116.7395, 368.7798) -> (156.8147, 340.1269) projected
  arc A60 (155.6515, 336.5) -> (156.8147, 340.1269) centre (155.6515, 338.5) ccw projected
  line L53 (155.6515, 336.5) -> (115.5763, 336.5) projected
  arc A61 (113.5763, 338.5) -> (115.5763, 336.5) centre (115.5763, 338.5) ccw projected
  arc A62 (288.4236, 53.5) -> (286.4236, 51.5) centre (288.4236, 51.5) ccw projected
  line L54 (288.4236, 53.5) -> (328.4988, 53.5) projected
  arc A63 (329.662, 49.8731) -> (328.4988, 53.5) centre (328.4988, 51.5) ccw projected
  line L55 (329.662, 49.8731) -> (289.5868, 21.2202) projected
  arc A64 (286.4236, 22.8472) -> (289.5868, 21.2202) centre (288.4236, 22.8472) ccw projected
  line L56 (286.4236, 22.8472) -> (286.4236, 51.5) projected
  arc A65 (115.5763, 53.5) -> (113.5763, 51.5) centre (115.5763, 51.5) ccw projected
  line L57 (115.5763, 53.5) -> (155.6515, 53.5) projected
  arc A66 (156.8147, 49.8731) -> (155.6515, 53.5) centre (155.6515, 51.5) ccw projected
  line L58 (156.8147, 49.8731) -> (116.7395, 21.2202) projected
  arc A67 (113.5763, 22.8472) -> (116.7395, 21.2202) centre (115.5763, 22.8472) ccw projected
  line L59 (113.5763, 22.8472) -> (113.5763, 51.5) projected
  line L60 (235, 259.9271) -> (235, 129.9271)
  line L61 (240.6723, 129.9271) -> (240.6723, 259.9271)
  line L62 (280, 73) -> (235, 73)
  line L63 (235, 73) -> (235, 317)
  line L64 (235, 317) -> (280, 317)
  line L65 (280, 317) -> (280, 73)
  point P0 (280, 129.9271)
  point P1 (280, 259.9271)
  dimension "d72" = 45
  constraints: 12 end point, 4 point on line, 3 perpendicular, 2 parallel, 1 horizontal
  measures "d72" distance between parallel lines of L8 L60
extrude "Выдавливание4" cut sketch "Эскиз4" against normal blind 10 contours L8 L62 L63 L3 | L3 L61 L1 L8 | L1 L63 L64 L8 | L3 L60 L1 L61
sketch "Эскиз5" plane through (0, 0, 0) normal (0, 0, -1) x (-1, 0, 0)
  line L0 (0, 390) -> (0, 0) projected
  line L1 (0, 390) -> (0, 0)
  line L2 (0, 195) -> (-157, 195)
  circle A0 centre (-157, 195) radius 4
  point P0 (0, 298)
  dimension "d75" = 157
  dimension "d76" = 8
  constraints: 4 end point, 1 centre point, 1 coincident, 1 horizontal, 1 midpoint, 1 vertical
  measures "d75" distance of L2.start L2.end
  measures "d76" diameter of A0
extrude "Выдавливание5" cut sketch "Эскиз5" against normal blind 10
